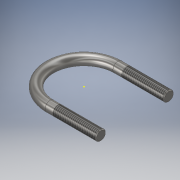
# Autodesk Inventor part: parafuso u abraçadeira
Saved by Autodesk Inventor 2019.4 (Build 234330000, 330)
## iProperties
Created: 2020-08-25
Part Number: parafuso u abraçadeira
Material: Aço inoxidável
Document SubType Name: Modeling
Designer: Lattes
Density: 8 g/cm^3
Appearance: Semipolido
Author: Lattes
Autodesk Inventor part; units mm, degrees
ref_plane "YZ Plane" through (0, 0, 0) normal (1, 0, 0) x (0, 1, 0)
ref_plane "XZ Plane" through (0, 0, 0) normal (0, 1, 0) x (-1, 0, 0)
ref_plane "XY Plane" through (0, 0, 0) normal (0, 0, 1) x (1, 0, 0)
sketch "Esboço1" plane through (0, 0, 0) normal (1, 0, 0) x (0, 1, 0)
  line L0 (0, 0) -> (15, 0)
  circle A0 centre (0, -20) radius 3
  constraints: 2 end point, 1 centre point, 1 horizontal
revolve "Revolução1" add sketch "Esboço1" angle 180 about axis through (0, 0, 0) along (0, 1, 0)
sketch "Esboço2" plane through (0, 0, 20) normal (1, 0, 0) x (0, 0, -1)
  circle A0 centre (0, 0) radius 3
  circle A1 centre (40, 0) radius 3
  point P0 (20, 0)
  constraints: 2 centre point
extrude "Extrusão1" add sketch "Esboço2" along normal blind 30
chamfer "Chanfro1" distance 0.5 angle 45 2 edges at (30, 0, -17) (30, 0, 23)
sketch "Esboço3" plane through (0, 0, 0) normal (0, 1, 0) x (-1, 0, 0)
  point P0 (0, 0)
thread "Rosca1" size "M6x1" class "6g" standard "ANSI Metric M Profile" length 25 offset 5
thread "Rosca2" size "M6x1" class "6g" standard "ANSI Metric M Profile" length 25
